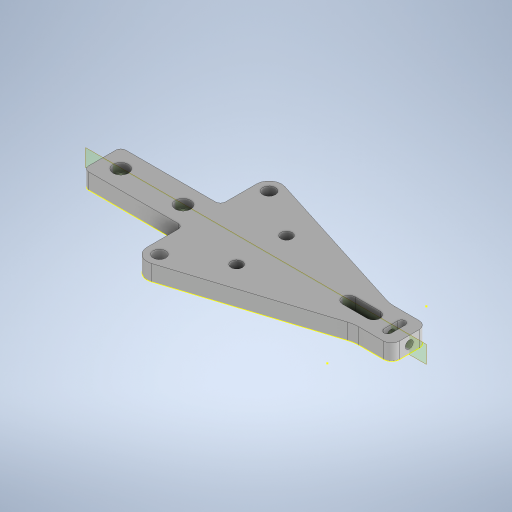
# Autodesk Inventor part: XZ Plate
Saved by Autodesk Inventor 2023.1 (Build 271208000, 208)
## iProperties
Created: 2022-10-29
Part Number: XZ Plate
Material: Generic
Document SubType Name: Modeling
Designer: nicol
Density: 1 g/cm^3
Appearance: Default
Author: nicol
Autodesk Inventor part; units mm, degrees
ref_plane "YZ Plane" through (0, 0, 0) normal (1, 0, 0) x (0, 1, 0)
ref_plane "XY Plane" through (0, 0, 0) normal (0, 0, 1) x (1, 0, 0)
sketch "Sketch1" plane through (0, 0, 0) normal (0, 0, 1) x (1, 0, 0)
  line L0 (-20, 150) -> (20, 150) construction
  line L1 (20, 150) -> (20, -150) construction
  line L2 (20, -150) -> (-20, -150) construction
  line L3 (-20, -150) -> (-20, 150) construction
  circle A0 centre (-30.5, 22) radius 11.95 construction
  circle A1 centre (-30.5, -22) radius 11.95 construction
  circle A2 centre (30.5, 0) radius 11.95 construction
  line L4 (42.45, 4.056) -> (42.45, -13.1126) construction
  circle A3 centre (30.5, 0) radius 7.5
  circle A4 centre (-30.5, 22) radius 5
  circle A5 centre (-30.5, -22) radius 5
  line L5 (-35.5, 3.8118) -> (-35.5, -3.8118) construction
  line L6 (0, 150) -> (0, -150) construction
  line L7 (-20, -108) -> (-20, -150) construction
  line L8 (-20, 150) -> (-20, 108) construction
  line L9 (-75.5, 7.5) -> (-35.5, 7.5)
  line L10 (-35.5, 7.5) -> (-35.5, -7.5)
  line L11 (-35.5, -7.5) -> (-75.5, -7.5)
  line L12 (-75.5, -7.5) -> (-75.5, 7.5)
  circle A6 centre (0, -150) radius 6 construction
  circle A7 centre (-11.5, -10) radius 4.5
  circle A8 centre (0, -150) radius 7
  line L13 (-7, -150) -> (-7, -10)
  line L14 (-11.5, 5.5) -> (-180, 5.5)
  line L15 (-11.5, -5.5) -> (-180, -5.5)
  line L16 (-185.5, -10) -> (-35.5, -10) construction
  line L17 (-35.5, -10) -> (-35.5, 10) construction
  line L18 (-35.5, 10) -> (-185.5, 10) construction
  line L19 (-185.5, 10) -> (-185.5, -10) construction
  circle A9 centre (-180, 0) radius 4.5 construction
  circle A10 centre (-180, 0) radius 5.5
  circle A11 centre (-11.5, -10) radius 2.5 construction
  line L20 (-35.5, -22) -> (-35.5, 22)
  line L21 (-28.9863, -26.7654) -> (32.7706, -7.148)
  line L22 (-28.9863, 26.7654) -> (32.7706, 7.148)
  line L23 (-20, 0) -> (0, 0)
  circle A12 centre (0, 150) radius 4.5 construction
  circle A13 centre (0, 150) radius 7
  line L24 (-7, 150) -> (-7, 10)
  circle A14 centre (-11.5, 10) radius 4.5
  line L25 (7, -150) -> (7, 150)
  point P0 (20, 0)
  point P1 (-29.8, 0)
  point P2 (-35.4948, -21.7719)
  point P3 (-35.4948, 21.7719)
  point P4 (-28.5008, 26.5829)
  point P5 (32.6594, 7.1824)
  point P6 (32.6594, -7.1824)
  point P7 (-28.5008, -26.5829)
  point P8 (-35.5, 0)
  point P9 (-68, 0)
  point P10 (-43, 0)
  point P11 (-75.5, 0)
  point P12 (-35.5, 0)
  point P13 (-95.75, -5.5)
  point P14 (-185.5, 0)
  dimension "d0" = 40
  dimension "d1" = 300
  dimension "d2" = 23.9
  dimension "d3" = 22
  dimension "d4" = 22
  dimension "d6" = 30.5
  dimension "d7" = 30.5
  dimension "d12" = 15
  dimension "d38" = 10
  dimension "d42" = 15
  dimension "d43" = 40
  dimension "d44" = 25
  dimension "d45" = 7.5
  dimension "d46" = 7.5
  dimension "d48" = 12
  dimension "d49" = 9
  dimension "d51" = 1
  dimension "d53" = 20
  dimension "d55" = 9
  dimension "d56" = 1
  dimension "d60" = 150
  dimension "d74" = 9
  dimension "d75" = 2.5
  dimension "d76" = 9
  constraints: 52 end point, 20 point on circle, 16 tangent, 14 centre point, 11 midpoint, 9 horizontal alignment, 7 parallel, 6 horizontal, 5 vertical, 4 collinear, 3 coincident, 3 equal radius, 3 perpendicular, 3 vertical alignment, 2 other
  measures "d0" distance of L0.start L0.end
  measures "d1" distance of L0.end L1.end
  measures "d2" diameter of A2
  measures "d3" vertical distance of L23.end A1.centre
  measures "d4" vertical distance of A0.centre L23.end
  measures "d6" distance of A2.centre L23.end
  measures "d7" horizontal distance of L23.end A0.centre
  measures "d12" diameter of A3
  measures "d38" diameter of A4
  measures "d42" distance of L11.end L9.start
  measures "d43" distance of L9.start L9.end
  measures "d44" distance of point (-43, 0) point (-68, 0)
  measures "d45" distance from line of L5 point (-43, 0)
  measures "d46" distance from line of L12 point (-68, 0)
  measures "d48" diameter of A6
  measures "d49" diameter of A7
  measures "d53" distance of L18.end L16.start
  measures "d55" diameter of A9
  measures "d56" radial gap between concentric circles of A9 A10
  measures "d60" distance of L17.end L18.end
  measures "d74" diameter of A12
  measures "d75" radial gap between concentric circles of A12 A13
  measures "d76" diameter of A14
extrude "Extrusion1" add sketch "Sketch1" against normal blind 6.35 contours A3 | A3 L21 L25 L22 | L25 L21 L13 A7 L15 L10 L14 A14 L24 L22 | L24 A14 L14 L10 L20 A4 L22 | L21 A5 L20 L10 L15 A7 L13 | A4 | A14 | A7 | A5 | L10 L14 L12 L9 | L10 L15 L12 L14 | L10 L11 L12 L15
hole "Hole1" at (-30.5, 22, 0) at (-30.5, -22, 0) at (30.5, 0, 0) direction (0, 0, -1) diameter 5.1 end through all
hole "Hole2" at (-43, 0, 0) at (-68, 0, 0) direction (0, 0, -1) diameter 3.2 end through all counterbore diameter 6.2 counterbore depth 3.58
fillet "Fillet1" radius 2 4 edges at (-75.5, 7.5, -3.175) (-75.5, -7.5, -3.175) (-35.5, -7.5, -3.175) (-35.5, 7.5, -3.175)
hole "Hole4" at (-11.5, -10, 0) at (-11.5, 10, 0) direction (0, 0, -1) diameter 4.5 end through all
sketch "Sketch3" plane through (0, 0, 0) normal (0, 0, 1) x (1, 0, 0)
  circle A0 centre (-11.5, -10) radius 2.25 projected
  circle A1 centre (-11.5, 10) radius 2.25 projected
  circle A2 centre (-43, 0) radius 3.1 projected
  circle A3 centre (-68, 0) radius 3.1 projected
  circle A4 centre (-30.5, 22) radius 2.55 projected
  circle A5 centre (-30.5, -22) radius 2.55 projected
  arc A6 (-75.5, -5.5) -> (-73.5, -7.5) centre (-73.5, -5.5) ccw projected
  line L0 (-73.5, -7.5) -> (-37.5, -7.5) projected
  arc A7 (-35.5, -9.5) -> (-37.5, -7.5) centre (-37.5, -9.5) ccw projected
  line L1 (-35.5, -9.5) -> (-35.5, -22) projected
  arc A8 (-35.5, -22) -> (-28.9863, -26.7654) centre (-30.5, -22) ccw projected
  line L2 (-28.9863, -26.7654) -> (32.7706, -7.148) projected
  arc A9 (32.7706, -7.148) -> (32.7706, 7.148) centre (30.5, 0) ccw projected
  line L3 (32.7706, 7.148) -> (-28.9863, 26.7654) projected
  arc A10 (-28.9863, 26.7654) -> (-35.5, 22) centre (-30.5, 22) ccw projected
  line L4 (-35.5, 22) -> (-35.5, 9.5) projected
  arc A11 (-37.5, 7.5) -> (-35.5, 9.5) centre (-37.5, 9.5) ccw projected
  line L5 (-37.5, 7.5) -> (-73.5, 7.5) projected
  arc A12 (-73.5, 7.5) -> (-75.5, 5.5) centre (-73.5, 5.5) ccw projected
  line L6 (-75.5, 5.5) -> (-75.5, -5.5) projected
  point P0 (0, 0)
  constraints: 1 coincident
sketch "Sketch4" plane through (0, 0, 0) normal (0, 0, 1) x (1, 0, 0)
  circle A0 centre (33.5, 0) radius 2.55 construction
  line L0 (33.5, 0) -> (23.5, 0) construction
  line L1 (33.5, 2.55) -> (23.5, 2.55)
  line L2 (23.5, -2.55) -> (33.5, -2.55)
  arc A1 (33.5, -2.55) -> (33.5, 2.55) centre (33.5, 0) ccw
  arc A2 (23.5, 2.55) -> (23.5, -2.55) centre (23.5, 0) ccw
  circle A3 centre (30.5, 0) radius 2.55 projected
  point P0 (0, 0)
  point P1 (28.5, 0)
  point P2 (33.5, 2.55)
  dimension "d78" = 10
  dimension "d97" = 3
  constraints: 8 end point, 4 point on circle, 4 tangent, 3 centre point, 1 concentric, 1 horizontal, 1 midpoint, 1 parallel, 1 point on line
  measures "d78" distance of L0.start L0.end
  measures "d97" distance of L0.start A3.centre
extrude "Extrusion2" cut sketch "Sketch4" against normal blind 25.4
sketch "Sketch5" plane through (0, 0, 0) normal (0, 0, 1) x (1, 0, 0)
  line L0 (32.7706, 7.148) -> (-28.9863, 26.7654) projected
  line L1 (32.7706, 7.148) -> (47.7706, 7.148)
  line L2 (47.7706, 7.148) -> (47.7706, -7.148)
  line L3 (47.7706, -7.148) -> (32.7706, -7.148)
  line L4 (-28.9863, -26.7654) -> (32.7706, -7.148) projected
  line L5 (40.4103, 2.8) -> (43.4103, 2.8)
  line L6 (43.4103, 2.8) -> (43.4103, -2.8)
  line L7 (43.4103, -2.8) -> (40.4103, -2.8)
  line L8 (40.4103, -2.8) -> (40.4103, 2.8)
  line L9 (36.05, 2.2796) -> (36.05, -2.3678) construction
  arc A0 (32.7706, -7.148) -> (32.7706, 7.148) centre (30.5, 0) ccw projected
  circle A1 centre (41.9103, 2.8) radius 1.5
  circle A2 centre (41.9103, -2.8) radius 1.5
  arc A3 (33.5, -2.55) -> (33.5, 2.55) centre (33.5, 0) ccw projected
  point P0 (0, 0)
  point P1 (32.7098, 0)
  point P2 (40.4103, 0)
  point P3 (43.4103, 2.8)
  point P4 (40.4103, 2.8)
  dimension "d81" = 3
  dimension "d82" = 5.6
  dimension "d83" = 15
  dimension "d84" = 4.3603
  dimension "d85" = 4.3603
  constraints: 17 end point, 3 midpoint, 3 perpendicular, 2 horizontal, 2 parallel, 2 tangent, 1 centre point, 1 horizontal alignment, 1 vertical, 3 other
  measures "d81" distance of L5.start L5.end
  measures "d82" distance of L5.end L6.end
  measures "d83" distance of L0.start L1.end
  measures "d84" distance between parallel lines of L8 L9
  measures "d85" distance between parallel lines of L2 L6
extrude "Extrusion3" add sketch "Sketch5" against normal up to surface (6.35 mm away)
sketch "Sketch6" plane through (47.7706, -7.148, 0) normal (1, 0, 0) x (0, 0, -1)
  line L0 (6.35, 14.2961) -> (6.35, 0) projected
  line L1 (0, 14.2961) -> (6.35, 14.2961) projected
  line L2 (0, 0) -> (0, 14.2961) projected
  line L3 (0, 0) -> (6.35, 0) projected
  point P0 (0, 7.148)
  point P1 (3.175, 7.148)
  point P2 (0, 7.148)
  point P3 (3.175, 14.2961)
  constraints: 2 midpoint, 1 horizontal alignment, 1 vertical alignment
hole "Hole5" at (47.7706, 0, -3.175) direction (-1, 0, 0) diameter 3.2 depth 25.4 tip angle 118
fillet "Fillet2" radius 12.7 2 edges at (32.7706, 7.148, -3.175) (32.7706, -7.148, -3.175)
fillet "Fillet3" radius 3.175 2 edges at (47.7706, -7.148, -3.175) (47.7706, 7.148, -3.175)
sketch "Sketch7" plane through (0, 0, -6.35) normal (0, 0, -1) x (-1, 0, 0)
  arc A0 (-43.4103, -2.8) -> (-40.4103, -2.8) centre (-41.9103, -2.8) ccw projected
  line L0 (-43.4103, -2.8) -> (-43.4103, 2.8) projected
  arc A1 (-40.4103, 2.8) -> (-43.4103, 2.8) centre (-41.9103, 2.8) ccw projected
  line L1 (-40.4103, 2.8) -> (-40.4103, -2.8) projected
  line L2 (-33.5, 2.55) -> (-23.5, 2.55) projected
  arc A2 (-23.5, -2.55) -> (-23.5, 2.55) centre (-23.5, 0) ccw projected
  line L3 (-23.5, -2.55) -> (-33.5, -2.55) projected
  circle A3 centre (30.5, 22) radius 2.55 projected
  circle A4 centre (30.5, -22) radius 2.55 projected
  circle A5 centre (68, 0) radius 1.6 projected
  circle A6 centre (43, 0) radius 1.6 projected
  arc A7 (-44.5956, 7.148) -> (-47.7706, 3.973) centre (-44.5956, 3.973) ccw projected
  line L4 (-47.7706, 3.973) -> (-47.7706, -3.973) projected
  arc A8 (-47.7706, -3.973) -> (-44.5956, -7.148) centre (-44.5956, -3.973) ccw projected
  line L5 (-44.5956, -7.148) -> (-34.7392, -7.148) projected
  arc A9 (-30.8944, -7.744) -> (-34.7392, -7.148) centre (-34.7392, -19.848) ccw projected
  line L6 (-30.8944, -7.744) -> (28.9863, -26.7654) projected
  arc A10 (28.9863, -26.7654) -> (35.5, -22) centre (30.5, -22) ccw projected
  line L7 (35.5, -22) -> (35.5, -9.5) projected
  arc A11 (37.5, -7.5) -> (35.5, -9.5) centre (37.5, -9.5) ccw projected
  line L8 (37.5, -7.5) -> (73.5, -7.5) projected
  arc A12 (73.5, -7.5) -> (75.5, -5.5) centre (73.5, -5.5) ccw projected
  line L9 (75.5, -5.5) -> (75.5, 5.5) projected
  arc A13 (75.5, 5.5) -> (73.5, 7.5) centre (73.5, 5.5) ccw projected
  line L10 (73.5, 7.5) -> (37.5, 7.5) projected
  arc A14 (35.5, 9.5) -> (37.5, 7.5) centre (37.5, 9.5) ccw projected
  line L11 (35.5, 9.5) -> (35.5, 22) projected
  arc A15 (35.5, 22) -> (28.9863, 26.7654) centre (30.5, 22) ccw projected
  line L12 (28.9863, 26.7654) -> (-30.8944, 7.744) projected
  arc A16 (-34.7392, 7.148) -> (-30.8944, 7.744) centre (-34.7392, 19.848) ccw projected
  line L13 (-34.7392, 7.148) -> (-44.5956, 7.148) projected
  circle A17 centre (11.5, 10) radius 2.25 projected
  circle A18 centre (11.5, -10) radius 2.25 projected
  arc A19 (-33.5, 2.55) -> (-33.5, -2.55) centre (-33.5, 0) ccw projected
  point P0 (0, 0)
equation "\"d4\" = d3"
equation "\"d7\" = d6"
equation "\"d46\" = d45"
equation "\"CAM_OFFSET\" = -0.508"
body "Solid1"
